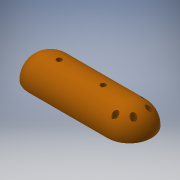
# Autodesk Inventor part: P1704_004_mainExterieur
Saved by Autodesk Inventor 2019 (Build 230136000, 136)
## iProperties
Created: 2019-05-02
Part Number: P1704_004_mainExterieur
Project: P1704 Manette
Material: PLA
Description: Main droite extérieur
Document SubType Name: Modeling
Designer: Joan.MAILLARD
Authority: brut Ø
Density: 1.25 g/cm^3
Appearance: Orange
Material number: ---
Author: Joan.MAILLARD
Title: P1704_004_mainDroiteExterieur
Autodesk Inventor part; units mm, degrees
ref_plane "Plan YZ" through (0, 0, 0) normal (1, 0, 0) x (0, 1, 0)
ref_plane "Plan XZ" through (0, 0, 0) normal (0, 1, 0) x (-1, 0, 0)
sketch "Esquisse1" plane through (0, 0, 0) normal (0, 0, 1) x (1, 0, 0)
  arc A0 (25, 25) -> (0, 0) centre (25, 0) ccw
  line L0 (25, 25) -> (115, 25)
  arc A1 (140, 0) -> (115, 25) centre (115, 0) ccw
  line L1 (0, 0) -> (140, 0)
  dimension "d0" = 90
  dimension "d1" = 25
  constraints: 5 point on circle, 4 end point, 2 centre point, 2 horizontal, 2 point on line, 2 tangent
  measures "d0" distance of L0.start L0.end
  measures "d1" distance from line of L1.start L0
revolve "Révolution1" add sketch "Esquisse1" angle 180 about axis through (0, 0, 0) along (1, 0, 0)
ref_plane "Plan de construction1" through (115, 25, 25) normal (0, 0, -1) x (-1, 0, 0)
sketch "Esquisse6" plane through (115, 25, 25) normal (0, 0, -1) x (-1, 0, 0)
  line L0 (76.7668, -25) -> (78.3834, -22.2)
  line L1 (78.3834, -22.2) -> (81.6166, -22.2)
  line L2 (81.6166, -22.2) -> (83.2332, -25)
  line L3 (83.2332, -25) -> (81.6166, -27.8)
  line L4 (81.6166, -27.8) -> (78.3834, -27.8)
  line L5 (78.3834, -27.8) -> (76.7668, -25)
  line L6 (90, 0) -> (90, -50) projected
  line L7 (26.7668, -25) -> (28.3834, -22.2)
  line L8 (28.3834, -22.2) -> (31.6166, -22.2)
  line L9 (31.6166, -22.2) -> (33.2332, -25)
  line L10 (33.2332, -25) -> (31.6166, -27.8)
  line L11 (31.6166, -27.8) -> (28.3834, -27.8)
  line L12 (28.3834, -27.8) -> (26.7668, -25)
  line L13 (30, -25) -> (26.7668, -25) construction
  line L14 (90, -25) -> (19.1163, -25) construction
  line L15 (80, -25) -> (76.7668, -25) construction
  point P0 (115, -25)
  dimension "d4" = 5.6
  dimension "d5" = 10
  dimension "d6" = 50
  dimension "d7" = 5.6
  constraints: 30 end point, 2 horizontal, 2 point on line, 1 collinear, 1 midpoint, 26 other
  measures "d4" distance between parallel lines of L3 L0
  measures "d5" distance from line of L6 L15.start
  measures "d6" distance of L13.start L15.start
  measures "d7" distance between parallel lines of L10 L7
extrude "Extrusion1" cut sketch "Esquisse6" along normal blind 12.5
sketch "Esquisse7" plane through (115, 25, 25) normal (0, 0, -1) x (-1, 0, 0)
  circle A0 centre (80, -25) radius 3.2332 construction
  circle A1 centre (30, -25) radius 3.2332 construction
  circle A2 centre (80, -25) radius 1.7
  circle A3 centre (30, -25) radius 1.7
  point P0 (115, -25)
  point P1 (78.3834, -22.2)
  point P2 (28.3834, -22.2)
  point P3 (31.6166, -27.8)
  point P4 (28.3834, -27.8)
  point P5 (81.6166, -27.8)
  point P6 (78.3834, -27.8)
  dimension "d10" = 3.4
  dimension "d11" = 3.4
  constraints: 6 point on circle, 4 centre point, 2 coincident
  measures "d10" diameter of A2
  measures "d11" diameter of A3
extrude "Extrusion2" cut sketch "Esquisse7" along normal blind 25
sketch "Esquisse8" plane through (115, 25, 25) normal (0, 0, -1) x (-1, 0, 0)
  line L0 (0.0645, -24.9628) -> (43.3013, 0) construction
  line L1 (43.3013, 0) -> (30.8013, 21.6506) construction
  line L2 (30.8013, 21.6506) -> (-34.1506, -15.8494) construction
  line L3 (-34.1506, -15.8494) -> (-21.6506, -37.5) construction
  line L4 (-21.6506, -37.5) -> (0.0645, -24.9628) construction
  arc A0 (0, 0) -> (0, -50) centre (0, -25) ccw projected
  line L5 (0, 0) -> (0, -50) projected
  line L6 (90, 0) -> (0, 0) projected
  line L7 (-0.0718, -8.8756) -> (-13.0622, -16.3756) construction
  circle A1 centre (-0.0718, -8.8756) radius 1.7
  circle A2 centre (-13.0622, -16.3756) radius 1.7
  line L8 (77.468, -25) -> (33.5617, -25) construction
  line L9 (55.5148, -25) -> (55.5148, 0) construction
  line L10 (55.5148, -25) -> (55.5148, -50) construction
  line L11 (0, -50) -> (90, -50) construction
  line L12 (-34.1506, -34.1506) -> (-21.6506, -12.5) construction
  line L13 (-21.6506, -12.5) -> (0.0645, -25.0372) construction
  arc A3 (0, 0) -> (0, -50) centre (0, -25) ccw
  line L14 (0, -50) -> (0, 0)
  line L15 (-0.0718, -41.1244) -> (-13.0622, -33.6244) construction
  circle A4 centre (-0.0718, -41.1244) radius 1.7
  circle A5 centre (-13.0622, -33.6244) radius 1.7
  point P0 (115, -25)
  dimension "d14" = 60
  dimension "d15" = 14
  dimension "d16" = 18
  dimension "d17" = 33
  dimension "d18" = 3.4
  dimension "d19" = 3.4
  constraints: 26 end point, 9 symmetric about line, 6 point on line, 5 centre point, 4 coincident, 4 perpendicular, 4 point on circle, 2 midpoint, 2 vertical, 1 collinear, 1 horizontal, 1 parallel, 1 tangent, 3 other
  measures "d14" angle of L5 L4
  measures "d15" distance between parallel lines of L0 L7
  measures "d16" distance from line of L7.end L3
  measures "d17" distance from line of L7.start L3
  measures "d18" diameter of A1
  measures "d19" diameter of A2
extrude "Extrusion3" cut sketch "Esquisse8" along normal blind 25 contours A1 L5 | L5 A1 | A4 L5 | L5 A4 | A2 | A5
sketch "Esquisse9" plane through (115, 25, 25) normal (0, 0, -1) x (-1, 0, 0)
  circle A0 centre (-0.0718, -8.8756) radius 3.25
  circle A1 centre (-13.0622, -16.3756) radius 3.25
  circle A2 centre (-0.0718, -8.8756) radius 1.7 projected
  circle A3 centre (-13.0622, -16.3756) radius 1.7 projected
  line L0 (67.152, -25) -> (35.9514, -25) construction
  line L1 (51.5517, -50) -> (51.5517, -25) construction
  line L2 (51.5517, -25) -> (51.5517, 0) construction
  line L3 (90, 0) -> (0, 0) construction
  line L4 (0, -50) -> (90, -50) construction
  circle A4 centre (-0.0718, -41.1244) radius 3.25
  circle A5 centre (-13.0622, -33.6244) radius 3.25
  circle A6 centre (-0.0718, -41.1244) radius 1.7
  circle A7 centre (-13.0622, -33.6244) radius 1.7
  point P0 (115, -25)
  dimension "d22" = 6.5
  dimension "d23" = 6.5
  constraints: 6 centre point, 6 end point, 4 symmetric about line, 2 concentric, 2 point on line, 2 vertical, 1 collinear, 1 horizontal, 1 midpoint, 4 other
  measures "d22" diameter of A0
  measures "d23" diameter of A1
extrude "Extrusion4" cut sketch "Esquisse9" along normal blind 12.5
equation "\"d7\" = d4"
equation "\"d11\" = d10"
equation "\"d19\" = d18"
equation "\"d23\" = d22"
